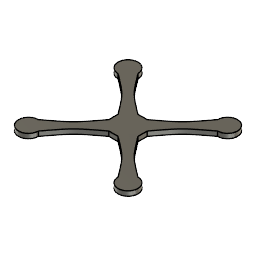
Drone 3 Polegadas (Autodesk Fusion 360 design; units mm, degrees)
Autodesk Fusion 360 part; units mm, degrees
sketch "Esboço1" plane through (0, 0, 0) normal (0, 0, 1) x (1, 0, 0)
  circle A0 centre (-53.1, 53.1) radius 10.65
  circle A1 centre (53.1, 53.1) radius 10.65
  circle A2 centre (-53.1, -53.1) radius 10.65
  circle A3 centre (53.1, -53.1) radius 10.65
  line L0 (0, 53.1) -> (0, -53.1) construction
  line L1 (-53.1, 0) -> (53.1, 0) construction
  line L2 (-53.1, -53.1) -> (-15.5526, -15.5526) construction
  line L3 (53.1, -53.1) -> (15.5526, -15.5526) construction
  line L4 (53.1, 53.1) -> (15.5526, 15.5526) construction
  line L5 (9.5526, -15.5526) -> (-9.5526, -15.5526)
  line L6 (-15.5526, -9.5526) -> (-15.5526, 9.5526)
  line L7 (-9.5526, 15.5526) -> (9.5526, 15.5526)
  line L8 (15.5526, 9.5526) -> (15.5526, -9.5526)
  line L9 (15.5526, -15.5526) -> (-15.5526, 15.5526) construction
  line L10 (-15.5526, -15.5526) -> (15.5526, 15.5526) construction
  line L11 (-42.45, 53.1) -> (-4.9431, 15.5526) construction
  line L12 (-53.1, 42.45) -> (-15.5526, 4.9026) construction
  line L13 (-23.6965, 34.3263) -> (-29.0114, 29.0114) construction
  line L14 (-34.3263, 23.6763) -> (-29.0114, 29.0114) construction
  spline S0 degree 2 poles (-42.45, 53.1) (-26.354, 31.6689) (-4.9431, 15.5526) knots 0 0 0 5.336996 5.336996 5.336996 weights 1 3 1
  spline S1 degree 2 poles (-53.1, 42.45) (-31.6689, 26.3439) (-15.5526, 4.9026) knots 0 0 0 5.339953 5.339953 5.339953 weights 1 3 1
  arc A4 (-9.5526, 15.5526) -> (-15.5526, 9.5526) centre (-9.5526, 9.5526) ccw
  spline S2 degree 2 poles (42.45, 53.1) (26.354, 31.6689) (4.9431, 15.5526) knots 0 0 0 5.336996 5.336996 5.336996 weights 1 3 1
  spline S3 degree 2 poles (53.1, 42.45) (31.6689, 26.3439) (15.5526, 4.9026) knots 0 0 0 5.339953 5.339953 5.339953 weights 1 3 1
  spline S4 degree 2 poles (-53.1, -42.45) (-31.6689, -26.3439) (-15.5526, -4.9026) knots 0 0 0 5.339953 5.339953 5.339953 weights 1 3 1
  spline S5 degree 2 poles (-42.45, -53.1) (-26.354, -31.6689) (-4.9431, -15.5526) knots 0 0 0 5.336996 5.336996 5.336996 weights 1 3 1
  spline S6 degree 2 poles (42.45, -53.1) (26.354, -31.6689) (4.9431, -15.5526) knots 0 0 0 5.336996 5.336996 5.336996 weights 1 3 1
  spline S7 degree 2 poles (53.1, -42.45) (31.6689, -26.3439) (15.5526, -4.9026) knots 0 0 0 5.339953 5.339953 5.339953 weights 1 3 1
  arc A5 (15.5526, 9.5526) -> (9.5526, 15.5526) centre (9.5526, 9.5526) ccw
  arc A6 (-15.5526, -9.5526) -> (-9.5526, -15.5526) centre (-9.5526, -9.5526) ccw
  arc A7 (9.5526, -15.5526) -> (15.5526, -9.5526) centre (9.5526, -9.5526) ccw
  dimension "d1" = 106.2
  dimension "d2" = 106.2
  dimension "d3" = 21.3
  dimension "d4" = 21.3
  dimension "d5" = 21.3
  dimension "d6" = 21.3
  dimension "d12" = 6
  dimension "d13" = 106.2
  dimension "d20" = 6
  dimension "d21" = 6
  dimension "d22" = 6
  constraint symmetric L0 A2.centre A3.centre
  constraint symmetric L0 L2.end L3.end
  constraint horizontal L5
  constraint perpendicular L5 L6
  constraint parallel L5 L7
  constraint parallel L6 L8
  constraint coincident L9 origin
  constraint coincident L10 origin
  constraint coincident A0 L11.start
  constraint coincident L7 L11.end
  constraint coincident A0 L12.start
  constraint coincident L6 L12.end
  constraint parallel L9 L12
  constraint midpoint L11 L13.start
  constraint midpoint L12 L14.start
  constraint coincident L9.end L7
  constraint coincident L9.end L6
  constraint tangent L7 A4
  constraint tangent L6 A4
  constraint symmetric L0 L11.start S2.start
  constraint symmetric L0 L11.end S2.end
  constraint symmetric L0 L12.start S3.start
  constraint symmetric L0 L12.end S3.end
  constraint symmetric L0 S0 S2
  constraint symmetric L0 S1 S3
  constraint symmetric L1 L11.start S5.start
  constraint symmetric L1 L11.end S5.end
  constraint symmetric L1 L12.start S4.start
  constraint symmetric L1 L12.end S4.end
  constraint symmetric L1 S0 S5
  constraint symmetric L1 S1 S4
  constraint symmetric L1 S2.start S6.start
  constraint symmetric L1 S2.end S6.end
  constraint symmetric L1 S2 S6
  constraint symmetric L1 S3.start S7.start
  constraint symmetric L1 S3.end S7.end
  constraint symmetric L1 S3 S7
  constraint coincident L4.end L7
  constraint coincident L4.end L8
  constraint tangent L7 A5
  constraint tangent L8 A5
  constraint coincident L2.end L6
  constraint coincident L2.end L5
  constraint tangent L6 A6
  constraint tangent L5 A6
  constraint coincident L3.end L5
  constraint coincident L3.end L8
  constraint tangent L5 A7
  constraint tangent L8 A7
  measures "d1" distance of A2.centre A3.centre
  measures "d2" distance of A0.centre A2.centre
  measures "d3" diameter of A0
  measures "d4" diameter of A1
  measures "d5" diameter of A2
  measures "d6" diameter of A3
  measures "d12" radius of A4
  measures "d13" distance of A0.centre A1.centre
  measures "d20" radius of A5
  measures "d21" radius of A6
  measures "d22" radius of A7
extrude "Extrusão1" add sketch "Esboço1" along normal blind 5
equation "d10 = 0.75"
equation "d11 = 0.75"
equation "d14 = d10"
equation "d15 = d11"
equation "d16 = d11"
equation "d17 = d10"
equation "d18 = d14"
equation "d19 = d15"
